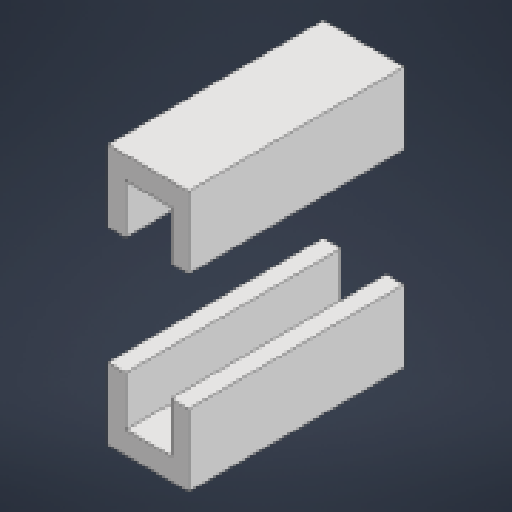
# Autodesk Inventor part: 2020_guide_adaptor
Saved by Autodesk Inventor 2024 (Build 280153000, 153)
## iProperties
Created: 2026-03-27
Part Number: 2020_guide_adaptor
Material: Generic
Document SubType Name: Modeling
Designer: schar
Density: 1 g/cm^3
Appearance: Default
Author: schar
Autodesk Inventor part; units mm, degrees
ref_plane "YZ Plane" through (0, 0, 0) normal (1, 0, 0) x (0, 1, 0)
ref_plane "XZ Plane" through (0, 0, 0) normal (0, 1, 0) x (-1, 0, 0)
ref_plane "XY Plane" through (0, 0, 0) normal (0, 0, 1) x (1, 0, 0)
sketch "Sketch3" plane through (0, 0, 0) normal (0, 0, 1) x (1, 0, 0)
  line L0 (0, 48) -> (-10, 48)
  line L1 (0, 42.5) -> (0, 48)
  line L2 (0, 5.5) -> (0, 42.5)
  line L3 (0, 0) -> (0, 5.5)
  line L4 (-10, 3) -> (0, 3)
  line L5 (-10, 5.5) -> (-10, 42.5)
  line L6 (-10, 5.5) -> (-10, 0)
  line L7 (-10, 48) -> (-10, 42.5)
  line L8 (0, 48) -> (-10, 48)
  line L9 (-10, 48) -> (-10, 53)
  line L10 (-10, 53) -> (0, 53)
  line L11 (0, 53) -> (0, 48)
  line L12 (-10, 3) -> (0, 3)
  line L13 (0, 3) -> (0, -2)
  line L14 (0, -2) -> (-10, -2)
  line L15 (-10, -2) -> (-10, 3)
  line L16 (-10, 53) -> (-14, 53)
  line L17 (-14, 53) -> (-14, 37)
  line L18 (-14, 37) -> (-10, 37)
  line L19 (-10, 37) -> (-10, 53)
  line L20 (0, 24) -> (-10, 24)
  line L21 (0, 53) -> (4, 53)
  line L22 (4, 53) -> (4, 37)
  line L23 (4, 37) -> (0, 37)
  line L24 (0, 37) -> (0, 53)
  line L25 (0, 0) -> (-10, 0)
  line L26 (0, 5.5) -> (0, 0)
  line L27 (-10, 0) -> (-10, 5.5)
  line L28 (0, 0) -> (-10, 0)
  line L29 (-10, 0) -> (-10, -5)
  line L30 (-10, -5) -> (0, -5)
  line L31 (0, -5) -> (0, 0)
  line L32 (-10, -5) -> (-14, -5)
  line L33 (-14, -5) -> (-14, 11)
  line L34 (-14, 11) -> (-10, 11)
  line L35 (-10, 11) -> (-10, -5)
  line L36 (0, -5) -> (4, -5)
  line L37 (4, -5) -> (4, 11)
  line L38 (4, 11) -> (0, 11)
  line L39 (0, 11) -> (0, -5)
extrude "Extrusion1" add sketch "Sketch3" against normal blind 48 contours L11 L21 L22 L23 L2 L1 | L0 L9 L10 L11 | L7 L5 L18 L17 L16 L9 | L38 L37 L36 L31 L13 L3 L2 | L5 L6 L15 L29 L32 L33 L34 | L13 L14 L15 L25 | L30 L29 L14 L31
sketch "Sketch4" plane through (4, -5, 0) normal (1, 0, 0) x (0, 0, -1)
  line L0 (22, 27) -> (22, 10) projected
  line L1 (26, 27) -> (26, 10) projected
  circle A0 centre (5.5, 10.5) radius 2.5 projected
  circle A1 centre (42.5, 10.5) radius 2.5 projected
  line L2 (22, 10) -> (26, 10) projected
  line L3 (-9.6, 29) -> (57.6, 29)
  line L4 (-9.6, 29) -> (57.6, 29)
  line L5 (22, 16.019) -> (20, 16.019)
  line L6 (20, 16.019) -> (20, 8.019)
  line L7 (26, 16.019) -> (28, 16.019)
  line L8 (28, 16.019) -> (28, 8.019)
  line L9 (28, 8.019) -> (20, 8.019)
  line L10 (20, 16.019) -> (28, 16.019)
  circle A2 centre (5.5, 47.5) radius 2.5
  circle A3 centre (42.5, 47.5) radius 2.5
  line L11 (20, 41.981) -> (20, 49.981)
  line L12 (28, 41.981) -> (28, 49.981)
  line L13 (28, 49.981) -> (20, 49.981)
  line L14 (20, 41.981) -> (28, 41.981)
  point P0 (0, 5)
  point P1 (26, 41.981)
  dimension "d8" = 2
  dimension "d9" = 8
  dimension "d10" = 2
  constraints: 24 end point, 7 symmetric about line, 5 horizontal, 3 perpendicular, 2 centre point, 2 point on line, 4 other
  measures "d8" distance of L5.start L5.end
  measures "d9" distance of L5.end L6.end
  measures "d10" distance of L7.start L7.end
extrude "Extrusion2" cut sketch "Sketch4" against normal through all
sketch "Sketch5" plane through (0, 0, 0) normal (0, 0, 1) x (1, 0, 0)
  line L0 (4, -5) -> (-14, -5) projected
  line L1 (-103.5812, 24) -> (13.5812, 24)
  line L2 (7.6307, 24) -> (-16.2188, 24)
  line L3 (-5, -5) -> (-5, -15)
  line L4 (0, -5) -> (0, -15)
  line L5 (0, -15) -> (-10, -15)
  line L6 (-10, -15) -> (-10, -5)
  line L7 (-10, -5) -> (0, -5)
  line L8 (0, -5) -> (-10, -15) construction
  line L9 (0, -15) -> (-10, -5) construction
  circle A0 centre (-5, -10) radius 2.5
  line L10 (0, -15) -> (4, -15)
  line L11 (4, -15) -> (4, -5)
  line L12 (4, -5) -> (0, -5)
  line L13 (0, -5) -> (0, -15)
  line L14 (-10, -15) -> (-14, -15)
  line L15 (-14, -15) -> (-14, -5)
  line L16 (-14, -5) -> (-10, -5)
  line L17 (-10, -5) -> (-10, -15)
  line L18 (4, 53) -> (-14, 53)
  line L19 (-5, 53) -> (-5, 63)
  line L20 (0, 53) -> (0, 63)
  line L21 (0, 63) -> (-10, 63)
  line L22 (-10, 63) -> (-10, 53)
  line L23 (-10, 53) -> (0, 53)
  line L24 (0, 53) -> (-10, 63) construction
  line L25 (0, 63) -> (-10, 53) construction
  circle A1 centre (-5, 58) radius 2.5
  line L26 (0, 63) -> (4, 63)
  line L27 (4, 63) -> (4, 53)
  line L28 (4, 53) -> (0, 53)
  line L29 (0, 53) -> (0, 63)
  line L30 (-10, 63) -> (-14, 63)
  line L31 (-14, 63) -> (-14, 53)
  line L32 (-14, 53) -> (-10, 53)
  line L33 (-10, 53) -> (-10, 63)
  point P0 (0, 0)
  dimension "d13" = 10
  dimension "d14" = 10
  dimension "d15" = 5
  constraints: 66 end point, 14 symmetric about line, 6 midpoint, 6 parallel, 3 horizontal, 3 perpendicular, 2 centre point, 2 coincident, 2 point on line, 2 vertical, 3 other
  measures "d13" distance of L3.start L3.end
  measures "d14" distance of L4.end L5.end
  measures "d15" diameter of A0
extrude "Extrusion3" add sketch "Sketch5" against normal blind 4 contours L11 L10 L4 L0 | L4 L5 L3 A0 L0 | L3 A0 L5 L6 L0 | L6 L14 L15 L0 | L18 L20 L26 L27 | L18 L19 A1 L21 L20 | L18 L22 L21 L19 A1 | L18 L31 L30 L22
sketch "Sketch6" plane through (0, 0, -4) normal (0, 0, -1) x (-1, 0, 0)
  line L0 (-4, -5) -> (-4, -15) projected
  line L1 (-4, -15) -> (0, -15)
  line L2 (0, -15) -> (0, -5)
  line L3 (0, -5) -> (-4, -5)
  line L4 (-4, -5) -> (-4, -15)
  line L5 (14, 11) -> (14, -15) projected
  line L6 (14, -5) -> (10, -5)
  line L7 (10, -5) -> (10, -15)
  line L8 (10, -15) -> (14, -15)
  line L9 (14, -15) -> (14, -5)
  line L10 (-13.5812, 24) -> (103.5812, 24)
  line L11 (-4, 53) -> (-4, 63)
  line L12 (-4, 63) -> (0, 63)
  line L13 (0, 63) -> (0, 53)
  line L14 (0, 53) -> (-4, 53)
  line L15 (14, 37) -> (14, 63)
  line L16 (14, 53) -> (10, 53)
  line L17 (10, 53) -> (10, 63)
  line L18 (10, 63) -> (14, 63)
  point P0 (0, 0)
  dimension "d18" = 4
  constraints: 34 end point, 11 symmetric about line, 6 point on line, 4 parallel, 3 horizontal, 2 perpendicular, 2 other
  measures "d18" distance of L8.end L7.end
extrude "Extrusion4" add sketch "Sketch6" along normal blind 10
sketch "Sketch7" plane through (4, -5, -48) normal (1, 0, 0) x (0, 0, -1)
  line L0 (-48, -10) -> (-34, -10) projected
  line L1 (-34, -10) -> (-44, -10)
  line L2 (-34, 0) -> (0, 0) projected
  line L3 (-44, -10) -> (-34, 0)
  line L4 (-34, 0) -> (-34, -10) projected
  line L5 (-34, -10) -> (-34, 0)
  line L6 (-34, 68) -> (-34, 58) projected
  line L7 (-34, 58) -> (-34, 68)
  line L8 (-34, 68) -> (-44, 68)
  line L9 (-44, 68) -> (-34, 58)
  point P0 (-48, 5)
  dimension "d21" = 10
  dimension "d22" = 10
  constraints: 12 end point, 1 collinear, 1 perpendicular, 1 point on line, 1 vertical
  measures "d21" distance of L0.end L1.end
  measures "d22" distance of L6.start L8.end
extrude "Extrusion5" cut sketch "Sketch7" against normal through all
body "Solid1"
